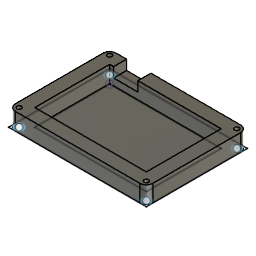
HackPad2 (Autodesk Fusion 360 design; units mm, degrees)
part number: 2025-12-24-22-20-42-012
part number: 2025-12-24-22-25-07-918
Autodesk Fusion 360 part; units mm, degrees
sketch "Sketch1" plane through (0, 0, 0) normal (0, 0, 1) x (1, 0, 0) in component "Adrian's HackPAd"
  line L0 (0, 0) -> (85, 0)
  line L1 (85, 0) -> (85, -57)
  line L2 (85, -57) -> (0, -57)
  line L3 (0, -57) -> (0, 0)
  line L4 (-10, -67) -> (95, -67)
  line L5 (95, -67) -> (95, 10)
  line L6 (95, 10) -> (-10, 10)
  line L7 (-10, 10) -> (-10, -67)
  circle A0 centre (-6, -63) radius 1.7
  circle A1 centre (-6, 6) radius 1.7
  circle A2 centre (91, -63) radius 1.7
  circle A3 centre (91, 6) radius 1.7
  circle A4 centre (-6, -63) radius 1.7
  circle A5 centre (-6.0108, -63.0177) radius 3
  circle A6 centre (-6.0108, -63.0177) radius 3
  circle A7 centre (-6.0108, -63.0177) radius 3
  circle A8 centre (-6.0108, 5.9294) radius 3
  circle A9 centre (91.0298, 5.9865) radius 3
  circle A10 centre (90.9857, -63.0067) radius 3
  dimension "d6" = 85
  dimension "d7" = 57
  dimension "d8" = 77
  dimension "d9" = 105
  dimension "d10" = 10
  dimension "d11" = 10
  dimension "d12" = 3.4
  dimension "d13" = 3.4
  dimension "d14" = 5.6569
  dimension "d15" = 5.6569
  dimension "d16" = 3.4
  dimension "d17" = 3.4
  dimension "d18" = 3.4
  dimension "d19" = 6
  dimension "d20" = 6
  dimension "d21" = 6
  dimension "d22" = 6
  dimension "d23" = 6
  dimension "d24" = 6
  constraint horizontal L0
  constraint vertical L1
  constraint horizontal L2
  constraint vertical L3
  constraint coincident L0.start L3.end
  constraint horizontal L4
  constraint vertical L5
  constraint horizontal L6
  constraint vertical L7
  measures "d6" distance of L0.start L0.end
  measures "d7" distance of L0.start L2.end
  measures "d8" distance of L4.start L6.end
  measures "d9" distance of L5.end L6.end
  measures "d10" horizontal distance of L1.end L4.end
  measures "d11" vertical distance of L0.start L6.end
  measures "d12" diameter of A0
  measures "d13" diameter of A1
  measures "d14" distance of L4.start A0.centre
  measures "d15" distance of L6.end A1.centre
  measures "d16" diameter of A2
  measures "d17" diameter of A3
  measures "d18" diameter of A4
  measures "d19" diameter of A5
  measures "d20" diameter of A6
  measures "d21" diameter of A7
  measures "d22" diameter of A8
  measures "d23" diameter of A9
  measures "d24" diameter of A10
extrude "Extrude1" add sketch "Sketch1" along normal blind 9.9 from surface at 3.1 contours A5 A6 A7 | A8 | A9 | A10 makes body 1 at (90.0303, -65.8504, 9.7) makes body 2 at (91.8423, 8.8744, 9.7) makes body 3 at (-8.1055, -65.1653, 9.7) makes body 4 at (-3.0145, 5.7798, 9.7) in component "Adrian's HackPAd"
extrude "Extrude2" add sketch "Sketch1" along normal blind 13 contours L4 L5 L6 L7 bodies 1 2 3 4 in component "Adrian's HackPAd"
extrude "Extrude3" add sketch "Sketch1" along normal blind 0.3 contours L0 L1 L2 L3 bodies 1 in component "Adrian's HackPAd"
sketch "Sketch2" plane through (0, 0, 13) normal (0, 0, 1) x (-1, 0, 0) in component "Adrian's HackPAd"
  circle A0 centre (-91, 63) radius 1.7
  circle A1 centre (6, -6) radius 1.7
  line L0 (-85, 57) -> (0, 57)
  line L1 (0, 57) -> (0, 0)
  line L2 (0, 0) -> (-85, 0)
  line L3 (-85, 0) -> (-85, 57)
  line L4 (10, -10) -> (10, 67)
  line L5 (10, 67) -> (-95, 67)
  line L6 (-95, 67) -> (-95, -10)
  line L7 (-95, -10) -> (10, -10)
  circle A2 centre (-91, -6) radius 1.7
  circle A3 centre (6, 63) radius 1.7
  line L8 (-3, -10) -> (-21.5, -10)
  line L9 (-21.5, -10) -> (-21.5, 0)
  line L10 (-21.5, 0) -> (-3, 0)
  line L11 (-3, 0) -> (-3, -10)
  line L12 (10, -10) -> (10, 67)
  dimension "d32" = 13
  dimension "d33" = 18.5
  constraint horizontal L8
  constraint vertical L9
  constraint horizontal L10
  constraint vertical L11
  constraint coincident L2 L9.end
  constraint coincident L7 L8.start
  measures "d32" distance of L10.end L12
  measures "d33" distance of L9.end L10.end
extrude "Extrude4" cut sketch "Sketch2" against normal blind 7.5 contours L2 L7 L8 L9 L10 L11 bodies 1 in component "Adrian's HackPAd"
fillet "Fillet1" radius 5 4 edges at (95, -67, 6.5) (95, 10, 6.5) (-10, -67, 6.5) (-10, 10, 6.5) on bodies 1 in component "Adrian's HackPAd"
component "Adrian's HackPAd" placed x (1, 0, 0) y (0, 1, 0) z (0, 0, 1) at (0, 0, 0)
